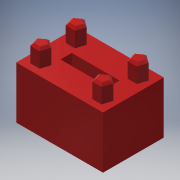
# Autodesk Inventor part: lego
Saved by Autodesk Inventor 2018.3 (Build 223284000, 284)
## iProperties
Created: 2020-11-17
Part Number: lego
Material: Generic
Document SubType Name: Modeling
Designer: Olivi
Density: 1 g/cm^3
Appearance: Light Red
Author: Olivi
Autodesk Inventor part; units mm, degrees
ref_plane "YZ Plane" through (0, 0, 0) normal (1, 0, 0) x (0, 1, 0)
ref_plane "XZ Plane" through (0, 0, 0) normal (0, 1, 0) x (-1, 0, 0)
ref_plane "XY Plane" through (0, 0, 0) normal (0, 0, 1) x (1, 0, 0)
sketch "Sketch1" plane through (0, 0, 0) normal (0, 0, 1) x (1, 0, 0)
  line L0 (0, 0) -> (20, 0)
  line L1 (20, 0) -> (20, 14)
  line L2 (20, 14) -> (0, 14)
  line L3 (0, 14) -> (0, 0)
  dimension "d0" = 20
  dimension "d1" = 14
  constraints: 8 end point, 2 parallel, 1 horizontal, 1 perpendicular
  measures "d0" distance of L2.end L1.end
  measures "d1" distance of L1.end L0.end
extrude "Extrusion1" add sketch "Sketch1" along normal blind 12
sketch "Sketch2" plane through (0, 0, 12) normal (0, 0, 1) x (1, 0, 0)
  line L0 (0, 0) -> (20, 0) projected
  line L1 (20, 14) -> (0, 14) projected
  line L2 (0, 14) -> (0, 0) projected
  line L3 (4.6094, 11.6352) -> (3.945, 9.5904)
  line L4 (3.945, 9.5904) -> (1.795, 9.5904)
  line L5 (1.795, 9.5904) -> (1.1306, 11.6352)
  line L6 (1.1306, 11.6352) -> (2.87, 12.8989)
  line L7 (2.87, 12.8989) -> (4.6094, 11.6352)
  line L8 (18.8694, 11.6352) -> (18.205, 9.5904)
  line L9 (18.205, 9.5904) -> (16.055, 9.5904)
  line L10 (16.055, 9.5904) -> (15.3906, 11.6352)
  line L11 (15.3906, 11.6352) -> (17.13, 12.8989)
  line L12 (17.13, 12.8989) -> (18.8694, 11.6352)
  line L13 (4.6094, 3.4952) -> (3.945, 1.4504)
  line L14 (3.945, 1.4504) -> (1.795, 1.4504)
  line L15 (1.795, 1.4504) -> (1.1306, 3.4952)
  line L16 (1.1306, 3.4952) -> (2.87, 4.7589)
  line L17 (2.87, 4.7589) -> (4.6094, 3.4952)
  line L18 (18.8694, 3.4952) -> (18.205, 1.4504)
  line L19 (18.205, 1.4504) -> (16.055, 1.4504)
  line L20 (16.055, 1.4504) -> (15.3906, 3.4952)
  line L21 (15.3906, 3.4952) -> (17.13, 4.7589)
  line L22 (17.13, 4.7589) -> (18.8694, 3.4952)
  point P0 (2.87, 11.07)
  point P1 (17.13, 11.07)
  point P2 (2.87, 2.93)
  point P3 (17.13, 2.93)
  dimension "d14" = 2.15
  dimension "d16" = 2.15
  dimension "d17" = 2.93
  dimension "d18" = 2.87
  dimension "d20" = 2.93
  dimension "d55" = 2.15
  dimension "d56" = 2.15
  constraints: 40 end point, 2 horizontal alignment, 2 vertical alignment, 1 parallel, 44 other
  measures "d14" distance of L14.start L14.end
  measures "d16" distance of L18.end L19.end
  measures "d17" distance from line of L1 point (2.87, 11.07)
  measures "d18" distance from line of L2 point (2.87, 11.07)
  measures "d20" distance from line of L0 point (2.87, 2.93)
  measures "d55" distance of L3.end L4.end
  measures "d56" distance of L9.start L9.end
extrude "Extrusion2" add sketch "Sketch2" along normal blind 4
chamfer "Chamfer1" distance 0.5 angle 45 20 edges at (4.2772, 10.6128, 16) (2.87, 9.5904, 16) (1.4628, 10.6128, 16) (2.0003, 12.267, 16) (3.7397, 12.267, 16) (3.7397, 4.127, 16) (2.0003, 4.127, 16) (1.4628, 2.4728, 16) (2.87, 1.4504, 16) (4.2772, 2.4728, 16) (17.13, 1.4504, 16) (15.7228, 2.4728, 16) (16.2603, 4.127, 16) (17.9997, 4.127, 16) (18.5372, 2.4728, 16) (17.13, 9.5904, 16) (18.5372, 10.6128, 16) (17.9997, 12.267, 16) (16.2603, 12.267, 16) (15.7228, 10.6128, 16)
sketch "Sketch3" plane through (0, 0, 0) normal (0, 0, -1) x (-1, 0, 0)
  line L0 (0, 0) -> (-20, 0) projected
  line L1 (0, 14) -> (0, 0) projected
  line L2 (-20, 14) -> (0, 14) projected
  line L3 (-20, 0) -> (-20, 14) projected
  line L4 (-4.8116, 3.5609) -> (-2.87, 4.9716)
  line L5 (-2.87, 4.9716) -> (-0.9284, 3.5609)
  line L6 (-0.9284, 3.5609) -> (-1.67, 1.2783)
  line L7 (-1.67, 1.2783) -> (-4.07, 1.2783)
  line L8 (-4.07, 1.2783) -> (-4.8116, 3.5609)
  line L9 (-19.0716, 3.5609) -> (-17.13, 4.9716)
  line L10 (-17.13, 4.9716) -> (-15.1884, 3.5609)
  line L11 (-15.1884, 3.5609) -> (-15.93, 1.2783)
  line L12 (-15.93, 1.2783) -> (-18.33, 1.2783)
  line L13 (-18.33, 1.2783) -> (-19.0716, 3.5609)
  line L14 (-2.87, 13.1116) -> (-0.9284, 11.7009)
  line L15 (-0.9284, 11.7009) -> (-1.67, 9.4183)
  line L16 (-1.67, 9.4183) -> (-4.07, 9.4183)
  line L17 (-4.07, 9.4183) -> (-4.8116, 11.7009)
  line L18 (-4.8116, 11.7009) -> (-2.87, 13.1116)
  line L19 (-17.13, 13.1116) -> (-15.1884, 11.7009)
  line L20 (-15.1884, 11.7009) -> (-15.93, 9.4183)
  line L21 (-15.93, 9.4183) -> (-18.33, 9.4183)
  line L22 (-18.33, 9.4183) -> (-19.0716, 11.7009)
  line L23 (-19.0716, 11.7009) -> (-17.13, 13.1116)
  point P0 (-2.87, 2.93)
  point P1 (-17.13, 2.93)
  point P2 (-2.87, 11.07)
  point P3 (-17.13, 11.07)
  dimension "d30" = 2.4
  dimension "d31" = 2.4
  dimension "d32" = 2.4
  dimension "d33" = 2.4
  dimension "d34" = 2.87
  dimension "d35" = 2.87
  dimension "d36" = 2.93
  dimension "d37" = 2.93
  constraints: 40 end point, 4 parallel, 2 horizontal alignment, 2 vertical alignment, 44 other
  measures "d30" distance of L19.start L19.end
  measures "d31" distance of L4.end L5.end
  measures "d32" distance of L9.end L10.end
  measures "d33" distance of L14.start L14.end
  measures "d34" distance from line of L1 point (-2.87, 2.93)
  measures "d35" distance from line of L3 point (-17.13, 2.93)
  measures "d36" distance from line of L0 point (-2.87, 2.93)
  measures "d37" distance from line of L2 point (-2.87, 11.07)
extrude "Extrusion3" cut sketch "Sketch3" against normal blind 4.5 contours L4 L5 L6 L7 L8 | L9 L10 L11 L12 L13 | L14 L15 L16 L17 L18 | L19 L20 L21 L22 L23
chamfer "Chamfer2" distance 0.5 angle 45 20 edges at (17.13, 1.2783, 0) (18.7008, 2.4196, 0) (15.5592, 2.4196, 0) (16.1592, 4.2662, 0) (18.1008, 4.2662, 0) (1.8992, 4.2662, 0) (1.2992, 2.4196, 0) (2.87, 1.2783, 0) (4.4408, 2.4196, 0) (3.8408, 4.2662, 0) (4.4408, 10.5596, 0) (2.87, 9.4183, 0) (1.2992, 10.5596, 0) (1.8992, 12.4062, 0) (3.8408, 12.4062, 0) (16.1592, 12.4062, 0) (15.5592, 10.5596, 0) (17.13, 9.4183, 0) (18.7008, 10.5596, 0) (18.1008, 12.4062, 0)
sketch "Sketch5" plane through (0, 0, 12) normal (0, 0, 1) x (1, 0, 0)
  line L0 (20, 14) -> (0, 14) projected
  line L1 (0, 14) -> (0, 0) projected
  line L2 (4.5, 8.3) -> (15.5, 8.3)
  line L3 (15.5, 8.3) -> (15.5, 5.7)
  line L4 (15.5, 5.7) -> (4.5, 5.7)
  line L5 (4.5, 5.7) -> (4.5, 8.3)
  dimension "d60" = 11
  dimension "d61" = 2.6
  dimension "d62" = 5.7
  dimension "d63" = 4.5
  constraints: 8 end point, 2 parallel, 1 horizontal, 1 perpendicular
  measures "d60" distance of L3.end L4.end
  measures "d61" distance of L2.end L3.end
  measures "d62" distance between parallel lines of L0 L2
  measures "d63" distance between parallel lines of L1 L5
extrude "Extrusion5" cut sketch "Sketch5" against normal up to next
body "Solid1"
